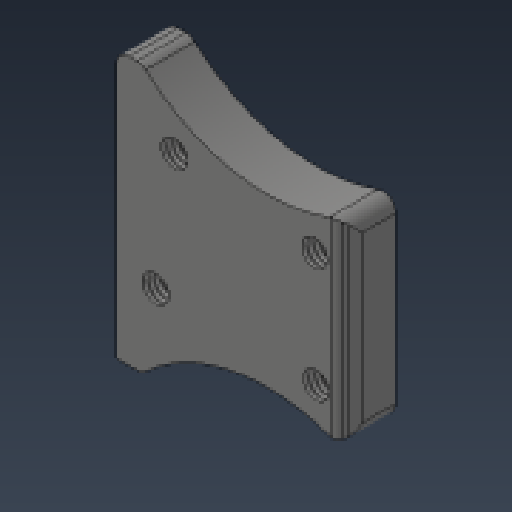
# Autodesk Inventor part: GearboxBearingHolderCover
Saved by Autodesk Inventor 2026.2 (Build 302298010, 298A)
## iProperties
Created: 2026-04-14
Part Number: GearboxBearingHolderCover
Material: Nylon 6/6
Document SubType Name: Modeling
Designer: szymo
Density: 1.13 g/cm^3
Appearance: Default(1)
Mass: 0.841862 g
Surface Area: 10.3759 cm^2
Volume: 0.74501 cm^3
Author: szymo
Autodesk Inventor part; units mm, degrees
ref_plane "YZ Plane" through (0, 0, 0) normal (1, 0, 0) x (0, 1, 0)
ref_plane "XZ Plane" through (0, 0, 0) normal (0, 1, 0) x (-1, 0, 0)
ref_plane "XY Plane" through (0, 0, 0) normal (0, 0, 1) x (1, 0, 0)
sketch "Sketch1" plane through (0, 0, 0) normal (0, 0, 1) x (1, 0, 0)
  line L0 (5, -24.795) -> (3, -24.795)
  line L1 (3, -24.795) -> (3, -45.542)
  line L2 (3, -45.542) -> (5, -45.542)
  circle A0 centre (14.7, -14.7) radius 14
  circle A1 centre (14.7, -55.6371) radius 14
  circle A2 centre (14.7, -14.7) radius 14.7 construction
  line L3 (0, -14.7) -> (0, -55.6371) construction
  circle A3 centre (14.7, -55.6371) radius 14.7 construction
  circle A4 centre (12.35, -35.2722) radius 5
  line L4 (20.85, -27.2769) -> (20.85, -43.0602)
  circle A5 centre (14.7, -14.7) radius 14.7 construction
  circle A6 centre (14.7, -14.7) radius 14 projected
  circle A7 centre (14.7, -55.6371) radius 14.7 construction
  circle A8 centre (14.7, -55.6371) radius 14 projected
  circle A9 centre (12.35, -35.2722) radius 3.2 construction
  circle A10 centre (12.35, -35.2722) radius 4.8 construction
  arc A11 (20.5375, -41.0138) -> (20.3662, -29.2939) centre (12.35, -35.2722) ccw projected
  line L5 (23.1, -65.8371) -> (23.1, -22.4365)
  arc A12 (20.5375, -41.0138) -> (19.1616, -37.1701) centre (18.4906, -39.5784) ccw projected
  line L6 (19.1616, -37.1701) -> (17.1665, -36.6142) projected
  arc A13 (17.1665, -36.6142) -> (17.1253, -33.79) centre (12.35, -35.2722) ccw projected
  line L7 (17.1253, -33.79) -> (19.1032, -33.1761) projected
  arc A14 (19.1032, -33.1761) -> (20.3662, -29.2939) centre (18.3622, -30.7885) ccw projected
  point P0 (0, 0)
  point P1 (20.85, -30.841)
  point P2 (20.85, -39.496)
  dimension "d0" = 3
  dimension "d2" = 3.5
  dimension "d5" = 10
  dimension "d6" = 2
  dimension "d7" = 2
  dimension "d22" = 20.747
  constraints: 12 end point, 5 coincident, 4 point on circle, 4 vertical, 3 centre point, 2 concentric, 2 horizontal alignment, 2 perpendicular, 2 point on line, 1 horizontal, 8 other
  measures "d0" distance between parallel lines of L3 L1
  measures "d2" distance edge to line of A4 L4
  measures "d5" diameter of A4
  measures "d6" distance of L0.start L0.end
  measures "d7" distance of L1.end L2.end
  measures "d22" distance of L0.end L1.end
ref_plane "Work Plane1" through (5.5618, -42.0604, 3.6) normal (0, 0, 1) x (0.7075365, 0.7066768, 0)
ref_plane "Work Plane2" through (5.5618, -42.0604, 3.6) normal (0, 0, 1) x (0.7075365, 0.7066768, 0)
ref_plane "Work Plane3" through (5.5618, -42.0604, 2.6) normal (0, 0, 1) x (0.7075365, 0.7066768, 0)
extrude "Extrusion1" add sketch "Sketch1" along normal blind 2.8 contours A0 L4 A11 A14 L7 A4 L6 A12 A1 L2 L1 L0 | L4 A14 A11 | A11 A12 L4 | L4 A12 L6 A4 L7 A14
sketch "Sketch2" plane through (3, -45.542, 2.8) normal (0, 0, 1) x (1, 0, 0)
  circle A0 centre (9.35, 10.2698) radius 5 projected
  line L0 (0, 0) -> (0, 20.747) projected
  line L1 (2, 0) -> (0, 0) projected
  arc A1 (17.85, 2.4818) -> (2, 0) centre (11.7, -10.095) ccw projected
  line L2 (17.85, 18.2652) -> (17.85, 2.4818) projected
  arc A2 (2, 20.747) -> (17.85, 18.2652) centre (11.7, 30.842) ccw projected
  line L3 (0, 20.747) -> (2, 20.747) projected
  line L4 (16.35, 16.396) -> (16.35, 7.741)
  point P0 (-3, 45.542)
  constraints: 2 end point, 1 vertical
extrude "Extrusion2" add sketch "Sketch2" along normal blind 1 contours A0 | L0 L3 A2 L2 A1 L1
sketch "Sketch3" plane through (3, -45.542, 0) normal (-1, 0, 0) x (0, 0, 1)
  line L0 (0, 20.747) -> (3.8, 20.747) projected
  line L1 (0, 20.747) -> (0, 0) projected
  line L2 (3.8, 10.3735) -> (0, 10.3735) construction
  circle A0 centre (1.9, 10.3735) radius 1.9
  line L3 (0, 15.2698) -> (0, 5.2698) projected
  line L4 (0, 0) -> (3.8, 0) projected
  line L5 (3.8, 20.747) -> (3.8, 0) projected
  point P0 (0, 45.542)
  dimension "d48" = 90
  constraints: 2 end point, 2 midpoint, 2 tangent, 1 centre point
  measures "d48" angle of L5 L2
hole "Hole1" at (3, -35.1685, 1.9) direction (1, 0, 0) diameter 2.013 depth 4.35 thread size "M2.5x0.45" class "6H" standard "ISO Metric profile"
chamfer "Chamfer2" distance 0.8 angle 45 1 edges at (20.85, -35.1685, 3.8) measured on face at (20.85, -35.1685, 3.3)
fillet "Fillet4" radius 1 7 edges at (20.85, -43.0602, 1.5) (20.85, -27.2769, 1.5) (5, -24.795, 1.9) (5, -45.542, 1.9) (3, -24.795, 1.9) (20.85, -35.1685, 3) (20.05, -35.1685, 3.8)
sketch "Sketch5" plane through (0, 0, 0) normal (0, 0, -1) x (-1, 0, 0)
  arc A0 (-19.1616, -37.1701) -> (-16.455, -41.0297) centre (-18.4906, -39.5784) ccw projected
  line L0 (-16.455, -41.0297) -> (-15.2527, -39.3434) projected
  arc A1 (-17.1665, -36.6142) -> (-15.2527, -39.3434) centre (-12.35, -35.2722) ccw projected
  line L1 (-17.1665, -36.6142) -> (-19.1616, -37.1701) projected
  circle A2 centre (-18.4906, -39.5784) radius 1.35 projected
  arc A3 (-16.285, -29.3972) -> (-19.1032, -33.1761) centre (-18.3622, -30.7885) ccw projected
  line L2 (-19.1032, -33.1761) -> (-17.1253, -33.79) projected
  arc A4 (-15.1325, -31.118) -> (-17.1253, -33.79) centre (-12.35, -35.2722) ccw projected
  line L3 (-15.1325, -31.118) -> (-16.285, -29.3972) projected
  circle A5 centre (-18.3622, -30.7885) radius 1.35 projected
  arc A6 (-6.2434, -31.7071) -> (-9.8413, -28.6611) centre (-7.5039, -29.5481) ccw projected
  line L4 (-9.8413, -28.6611) -> (-10.5761, -30.5975) projected
  arc A7 (-8.032, -32.7513) -> (-10.5761, -30.5975) centre (-12.35, -35.2722) ccw projected
  line L5 (-8.032, -32.7513) -> (-6.2434, -31.7071) projected
  circle A8 centre (-7.5039, -29.5481) radius 1.35 projected
  arc A9 (-8.029, -40.8694) -> (-5.1631, -37.0044) centre (-6.0501, -39.3417) ccw projected
  line L6 (-5.1631, -37.0044) -> (-7.4268, -36.1454) projected
  arc A10 (-9.2946, -39.2301) -> (-7.4268, -36.1454) centre (-12.35, -35.2722) ccw projected
  line L7 (-9.2946, -39.2301) -> (-8.029, -40.8694) projected
  circle A11 centre (-6.0501, -39.3417) radius 1.35 projected
  point P0 (0, 0)
hole "Hole2" at (18.4906, -39.5784, 0) at (18.3622, -30.7885, 0) at (7.5039, -29.5481, 0) at (6.0501, -39.3417, 0) direction (0, 0, 1) diameter 2.013 end through all thread size "M2.5x0.45" class "6H" standard "ISO Metric profile"
equation "\"d7\" = d6"
body "Solid1"
